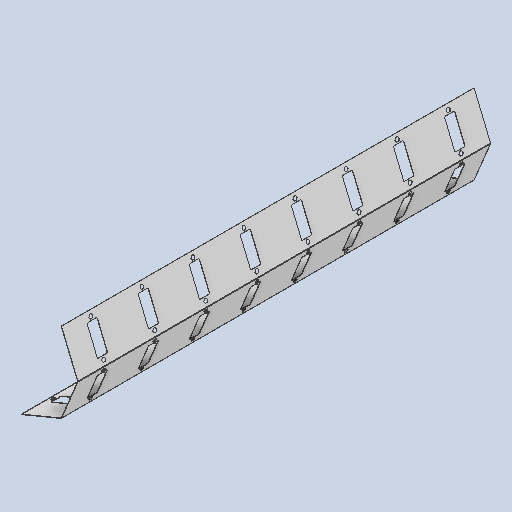
# Autodesk Inventor part: ДМФ 01 14 Барабан Лист прав брт v2.0
Saved by Autodesk Inventor 2025 (Build 290162010, 162A)
## iProperties
Created: 2024-04-28
Part Number: ДМФ 01 14 Барабан Лист прав брт v2.0
Material: Generic
Document SubType Name: Sheet Metal
Designer: pokla
Density: 1 g/cm^3
Appearance: Default
Sheet Metal Rule: Default
Flat Pattern Width: 63.3571 cm
Flat Pattern Length: 202 cm
Flat Pattern Area: 12798.1 cm^2
Sheet Metal Width: 633,571 mm
Sheet Metal Length: 2020,000 mm
Sheet Metal Area: 1279813,721 mm^2
Stock Number: Барабан_Лист_Правый_Борт
Author: pokla
Autodesk Inventor part; units mm, degrees
ref_plane "YZ Plane" through (0, 0, 0) normal (1, 0, 0) x (0, 1, 0)
ref_plane "XZ Plane" through (0, 0, 0) normal (0, 1, 0) x (-1, 0, 0)
ref_plane "XY Plane" through (0, 0, 0) normal (0, 0, 1) x (1, 0, 0)
sketch "Sketch2" plane through (0, 0, 0) normal (0, 0, 1) x (1, 0, 0)
  line L0 (0, 277.633599) -> (196.316601, 196.316601) construction
  line L1 (196.316601, 196.316601) -> (277.633599, 0) construction
  line L2 (277.633599, 0) -> (196.316601, -196.316601) construction
  line L3 (196.316601, -196.316601) -> (0, -277.633599) construction
  line L4 (0, -277.633599) -> (-196.316601, -196.316601) construction
  line L5 (-196.316601, -196.316601) -> (-277.633599, 0) construction
  line L6 (-277.633599, 0) -> (-196.316601, 196.316601) construction
  line L7 (-196.316601, 196.316601) -> (0, 277.633599) construction
  line L8 (196.661016, 195.485109) -> (276.999549, 1.530734)
  line L9 (276.999549, -1.530734) -> (196.950651, -194.785867)
  arc A0 (276.999549, -1.530734) -> (276.999549, 1.530734) centre (273.304031, 0) ccw
  line L10 (194.785867, -196.950651) -> (0.831492, -277.289184)
  arc A1 (194.785867, -196.950651) -> (196.950651, -194.785867) centre (193.255133, -193.255133) ccw
  point P0 (0, 0)
  point P1 (0, 0)
  dimension "d56" = 513
  dimension "d58" = 4
  dimension "d69" = 0.9
  dimension "d70" = 4
  dimension "d71" = 0.9
  measures "d56" distance between parallel lines of L6 L2
  measures "d58" radius of A0
  measures "d69" distance of L3.end L10.end
  measures "d70" radius of A1
  measures "d71" distance of L0.end L8.start
contour flange "Contour Flange2" sketch "Sketch2" thickness 2 bend radius 2 width 2020 along (0, 0, -1) mid plane no both sides no wall seen from (236.830282, 98.507921, 0) lies toward (-0.9238795, -0.3826834, 0) curves L8 A0 L9 A1 L10
bend "Bend2"
corner "Corner2"
sketch "Sketch10" plane through (196.950651, -194.785867, 0) normal (0.9238795, -0.3826834, 0) x (0, 0, -1)
  line L0 (1110, 172.088924) -> (1160, 172.088924)
  line L1 (1160, 172.088924) -> (1160, 37.088924)
  line L2 (1160, 37.088924) -> (1110, 37.088924)
  line L3 (1110, 37.088924) -> (1110, 172.088924)
  line L4 (1110, 104.588924) -> (1160, 104.588924) construction
  line L5 (2020, 209.177849) -> (2020, 0) construction
  line L6 (2020, 209.177849) -> (0, 209.177849) construction
  line L7 (1135, 187.088924) -> (1135, 22.088924) construction
  line L8 (1130.150258, 178.688924) -> (1125.300515, 187.088924)
  line L9 (1125.300515, 187.088924) -> (1130.150258, 195.488924)
  line L10 (1130.150258, 195.488924) -> (1139.849742, 195.488924)
  line L11 (1139.849742, 195.488924) -> (1144.699485, 187.088924)
  line L12 (1144.699485, 187.088924) -> (1139.849742, 178.688924)
  line L13 (1139.849742, 178.688924) -> (1130.150258, 178.688924)
  line L14 (1139.849742, 30.488924) -> (1144.699485, 22.088924)
  line L15 (1144.699485, 22.088924) -> (1139.849742, 13.688924)
  line L16 (1139.849742, 13.688924) -> (1130.150258, 13.688924)
  line L17 (1130.150258, 13.688924) -> (1125.300515, 22.088924)
  line L18 (1125.300515, 22.088924) -> (1130.150258, 30.488924)
  line L19 (1130.150258, 30.488924) -> (1139.849742, 30.488924)
  point P0 (0, 104.588924)
  point P1 (1135, 172.088924)
  point P2 (2020, 104.588924)
  point P3 (1010, 209.177849)
  point P4 (1010, 209.177849)
  point P5 (1135, 104.588924)
  point P6 (1135, 178.688924)
  point P7 (1135, 30.488924)
  dimension "d107" = 135
  dimension "d108" = 50
  dimension "d118" = 125
  dimension "d125" = 165
  dimension "d126" = 16.8
  dimension "d127" = 16.8
  constraints: 36 end point, 10 midpoint, 2 coincident, 2 parallel, 2 point on line, 1 horizontal, 1 horizontal alignment, 1 perpendicular, 1 vertical, 26 other
  measures "d107" distance of L0.end L1.end
  measures "d108" distance of L0.start L0.end
  measures "d118" horizontal distance of point (1010, 209.178) point (1135, 172.089)
  measures "d125" distance of L7.start L7.end
  measures "d126" distance between parallel lines of L13 L10
  measures "d127" distance between parallel lines of L16 L19
extrude "Extrusion4" cut sketch "Sketch10" against normal up to surface (2 mm away)
fillet "Fillet1" radius 5 4 edges at (261.8824, -35.4137, -1160) (261.8824, -35.4137, -1110) (210.2201, -160.1375, -1110) (210.2201, -160.1375, -1160)
pattern_circular "Circular Pattern1" count 3 over 90 about axis through (0, 0, -10) along (0, 0, 1) of "Extrusion4", "Fillet1" both ways yes
pattern_linear "Rectangular Pattern2" count 8 spacing 250 along (0, 0, 1) of "Extrusion4", "Fillet1", "Circular Pattern1" first direction both ways yes
chamfer "Corner Chamfer1" distance 2 angle 45 1 edges at (195.7371, 195.1024, -2020)
equation "\"d118\" = Барабан_Отступ_окна_от_середины"
equation "\"d56\" = Барабан_габарит_по_кассетам"
equation "\"d58\" = BendRadius + Thickness"
equation "\"d69\" = Барабан_отступ_развертки"
equation "\"d70\" = BendRadius + Thickness"
equation "\"d71\" = Барабан_отступ_развертки"
equation "\"d107\" = Барабан_Длина_окна"
equation "\"d108\" = Барабан_Ширина_окна"
equation "\"d25\" = Thickness"
equation "\"d26\" = BendReliefWidth"
equation "\"d27\" = BendReliefDepth"
equation "\"d28\" = MinimumRemnant"
equation "\"d29\" = TransitionRadius"
equation "\"d30\" = Барабан_длина_листа"
equation "\"d31\" = BendRadius"
equation "\"d33\" = CornerReliefSize"
equation "\"d34\" = GapSize"
equation "\"d35\" = JacobiRadiusSize"
equation "\"BendRadius\" = Thickness"
equation "\"BendReliefWidth\" = Thickness"
equation "\"BendReliefDepth\" = 0.5 * Thickness"
equation "\"CornerReliefSize\" = 4 * Thickness"
equation "\"MinimumRemnant\" = 2 * Thickness"
equation "\"TransitionRadius\" = BendRadius"
equation "\"JacobiRadiusSize\" = BendRadius"
equation "\"GapSize\" = Thickness"
equation "\"Барабан_габарит_по_кассетам\" = 513"
equation "\"Thickness\" = 2"
equation "\"Барабан_отступ_развертки\" = 0.9"
equation "\"Барабан_Длина_окна\" = 135"
equation "\"Барабан_Ширина_окна\" = 50"
equation "\"Барабан_длина_листа\" = 2020"
equation "\"Барабан_Отступ_окна_от_середины\" = 125"
body "Solid2"
